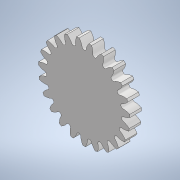
# Autodesk Inventor part: Pinion222
Saved by Autodesk Inventor 2022 (Build 260153000, 153)
## iProperties
Created: 2022-06-04
Part Number: Pinion222
Material: Generic
Document SubType Name: Modeling
Designer: frede
Density: 1 g/cm^3
Appearance: Default
Author: frede
Autodesk Inventor part; units mm, degrees
ref_plane "YZ Plane" through (0, 0, 0) normal (1, 0, 0) x (0, 1, 0)
ref_plane "XZ Plane" through (0, 0, 0) normal (0, 1, 0) x (-1, 0, 0)
ref_plane "XY Plane" through (0, 0, 0) normal (0, 0, 1) x (1, 0, 0)
sketch "Sketch1" plane through (0, 0, 0) normal (0, 0, 1) x (1, 0, 0)
  spline S0 degree 3 poles (-3.3489, 31.0344) (-3.2669, 30.9208) (-3.1027, 30.6937) (-2.8692, 30.344) (-2.6455, 29.988) (-2.4333, 29.625) (-2.2335, 29.255) (-2.0474, 28.8779) (-1.8767, 28.4936) (-1.7233, 28.102) (-1.5918, 27.7027) (-1.4824, 27.296) (-1.4363, 26.9482) (-1.3713, 26.6753) (-1.3031, 26.4761) (-1.2148, 26.2851) (-1.1055, 26.1048) (-0.9893, 25.973) (-0.8874, 25.8765) (-0.8022, 25.8147) (-0.714, 25.7572) (-0.6186, 25.7128) (-0.5212, 25.6728) (-0.4188, 25.6481) (-0.3154, 25.6283) (-0.1751, 25.6229) (0, 25.6264) (0.1751, 25.6229) (0.3154, 25.6283) (0.4188, 25.6481) (0.5212, 25.6728) (0.6186, 25.7128) (0.714, 25.7572) (0.8022, 25.8147) (0.8874, 25.8765) (0.9893, 25.973) (1.1055, 26.1048) (1.2148, 26.2851) (1.3031, 26.4761) (1.3713, 26.6753) (1.4363, 26.9482) (1.4824, 27.296) (1.5918, 27.7027) (1.7233, 28.102) (1.8767, 28.4936) (2.0474, 28.8779) (2.2335, 29.255) (2.4333, 29.625) (2.6455, 29.988) (2.8692, 30.344) (3.1027, 30.6937) (3.2669, 30.9208) (3.3489, 31.0344) knots 0 0 0 0 0.042039 0.084079 0.126119 0.168158 0.210197 0.252236 0.294274 0.336311 0.378346 0.420376 0.46241 0.483428 0.504444 0.525453 0.546459 0.567453 0.577965 0.588475 0.598984 0.609494 0.620001 0.63051 0.641019 0.651526 0.672547 0.693567 0.704074 0.714583 0.725092 0.735599 0.746109 0.756618 0.767128 0.77764 0.798635 0.81964 0.840649 0.861665 0.882683 0.924717 0.966747 1.008782 1.050819 1.092857 1.134896 1.176935 1.218975 1.261014 1.303054 1.345093 1.345093 1.345093 1.345093
  circle A0 centre (0, 0) radius 25.625 construction
  circle A1 centre (0, 0) radius 27.0162 construction
  circle A2 centre (0, 0) radius 28.75 construction
  circle A3 centre (0, 0) radius 31.2146
  point P0 (-3.1048, 30.6922)
  point P1 (-2.8708, 30.3429)
  point P2 (-2.6474, 29.9868)
  point P3 (-2.4354, 29.6238)
  point P4 (-2.2358, 29.2538)
  point P5 (-2.05, 28.8767)
  point P6 (-1.8796, 28.4924)
  point P7 (-1.7269, 28.1007)
  point P8 (-1.5955, 27.7015)
  point P9 (-1.4914, 27.2943)
  point P10 (-1.4177, 26.8804)
  point P11 (-1.368, 26.6762)
  point P12 (-1.2997, 26.4774)
  point P13 (-1.2113, 26.2869)
  point P14 (-1.1005, 26.1085)
  point P15 (-0.9631, 25.9497)
  point P16 (-0.8859, 25.8783)
  point P17 (-0.8017, 25.8154)
  point P18 (-0.7128, 25.7594)
  point P19 (-0.6182, 25.7135)
  point P20 (-0.5203, 25.6754)
  point P21 (-0.4186, 25.6489)
  point P22 (-0.3151, 25.6309)
  point P23 (-0.2102, 25.6249)
  point P24 (0, 25.625)
  point P25 (0.2102, 25.6249)
  point P26 (0.3151, 25.6309)
  point P27 (0.4186, 25.6489)
  point P28 (0.5203, 25.6754)
  point P29 (0.6182, 25.7135)
  point P30 (0.7128, 25.7594)
  point P31 (0.8017, 25.8154)
  point P32 (0.8859, 25.8783)
  point P33 (0.9631, 25.9497)
  point P34 (1.1005, 26.1085)
  point P35 (1.2113, 26.2869)
  point P36 (1.2997, 26.4774)
  point P37 (1.368, 26.6762)
  point P38 (1.4177, 26.8804)
  point P39 (1.4914, 27.2943)
  point P40 (1.5955, 27.7015)
  point P41 (1.7269, 28.1007)
  point P42 (1.8796, 28.4924)
  point P43 (2.05, 28.8767)
  point P44 (2.2358, 29.2538)
  point P45 (2.4354, 29.6238)
  point P46 (2.6474, 29.9868)
  point P47 (2.8708, 30.3429)
  point P48 (3.1048, 30.6922)
  constraints: 4 centre point, 2 point on circle, 107 other
extrude "Extrusion1" add sketch "Sketch1" against normal blind 8
extrude "Extrusion2" cut sketch "Sketch1" against normal through all contours A3 S0 picked at (-0.4102, 29.7407)
pattern_circular "Circular Pattern1" count 23 over 360 about axis through (0, 0, 0) along (0, 0, -1) of "Extrusion2"
sketch "Sketch2" plane through (0, 0, 0) normal (0, 0, 1) x (1, 0, 0)
  arc A0 (-47.6633, 66.2169) -> (-53.0859, 65.6856) centre (-50.338, 65.578) ccw projected
  line L0 (-53.0859, 65.6856) -> (-53.5665, 53.4075) projected
  arc A1 (-53.5665, 53.4075) -> (-52.7565, 45.1423) centre (-48.7825, 49.704) ccw projected
  line L1 (-52.7565, 45.1423) -> (-49.9016, 33.1911) projected
  arc A2 (-49.9016, 33.1911) -> (-44.479, 33.7225) centre (-47.2269, 33.8301) ccw projected
  line L2 (-44.479, 33.7225) -> (-43.9985, 46.0006) projected
  arc A3 (-43.9985, 46.0006) -> (-44.8084, 54.2658) centre (-48.7825, 49.704) ccw projected
  line L3 (-44.8084, 54.2658) -> (-47.6633, 66.2169) projected
  circle A4 centre (-48.7825, 49.704) radius 4.4 projected
  circle A5 centre (-48.0998, 42.7374) radius 0.75 projected
  circle A6 centre (-47.8072, 39.7517) radius 0.75 projected
  circle A7 centre (-47.5146, 36.766) radius 0.75 projected
  circle A8 centre (-50.3429, 65.6278) radius 0.75 projected
  circle A9 centre (-50.0503, 62.6421) radius 0.75 projected
  circle A10 centre (-49.7577, 59.6564) radius 0.75 projected
  circle A11 centre (-47.222, 33.7803) radius 0.75 projected
  circle A12 centre (-49.4651, 56.6707) radius 0.75 projected
  arc A13 (1.1192, 16.5129) -> (-4.3035, 15.9815) centre (-1.5556, 15.874) ccw
  line L4 (-4.3035, 15.9815) -> (-4.784, 3.7035)
  arc A14 (-4.784, 3.7035) -> (-3.974, -4.5617) centre (0, 0) ccw
  line L5 (-3.974, -4.5617) -> (-1.1192, -16.5129)
  arc A15 (4.784, -3.7035) -> (3.974, 4.5617) centre (0, 0) ccw
  line L6 (3.974, 4.5617) -> (1.1192, 16.5129)
  arc A16 (-1.1192, -16.5129) -> (4.3035, -15.9815) centre (1.5556, -15.874) ccw
  line L7 (4.3035, -15.9815) -> (4.784, -3.7035)
  line L8 (-3.974, -4.5617) -> (-1.1192, -16.5129)
  line L9 (-1.6055, -16.6291) -> (-4.424, -4.8302)
  arc A17 (-5.2775, 3.8795) -> (-4.424, -4.8302) centre (0, 0) ccw
  line L10 (-5.2775, 3.8795) -> (-4.8031, 16.0011)
  arc A18 (1.6055, 16.6291) -> (-4.8031, 16.0011) centre (-1.5556, 15.874) ccw
  line L11 (1.6055, 16.6291) -> (4.424, 4.8302)
  arc A19 (5.1794, -4.0096) -> (4.424, 4.8302) centre (0, 0) ccw
  line L12 (5.2836, -3.723) -> (4.8031, -16.0011)
  arc A20 (-1.6055, -16.6291) -> (4.8031, -16.0011) centre (1.5556, -15.874) ccw
  point P0 (-1.1192, -16.5129)
  point P1 (4.784, -3.7035)
  point P2 (1.1192, 16.5129)
  point P3 (5.2775, -3.8795)
  dimension "d9" = 360
  dimension "d13" = 0.5
  dimension "d14" = 0.5
  dimension "d15" = 0.5
  constraints: 18 end point, 16 point on circle, 8 centre point, 2 coincident, 24 other
  measures "d13" distance between parallel lines of L4 L10
  measures "d14" distance between parallel lines of L6 L11
  measures "d15" distance between parallel lines of L7 L12
extrude "Extrusion3" cut sketch "Sketch2" against normal blind 2.5 contours L6 A15 L7 A16 L5 A14 L4 A13 | L9 A17 L10 A18 L11 A19 L12 A20
sketch "Sketch3" plane through (0, 0, 0) normal (0, 0, 1) x (1, 0, 0)
  circle A0 centre (0, 0) radius 2
  dimension "d16" = 4
  constraints: 1 centre point, 1 coincident
  measures "d16" diameter of A0
extrude "Extrusion4" cut sketch "Sketch3" against normal through all
equation "\"d0\" = FaceWidth"
equation "\"Module\" = 2.5"
equation "\"PressureAngle\" = 20deg"
equation "\"UnitProfileClearance\" = 0.25"
equation "\"UnitRoundRadius\" = 0.35"
equation "\"HeadDiameter\" = 62.42917"
equation "\"RootDiameter\" = 51.25"
equation "\"BaseDiameter\" = 54.03233"
equation "\"PitchDiameter\" = 57.5"
equation "\"FaceWidth\" = 8"
equation "\"HelixAngle\" = 0"
equation "\"UnitCorrection\" = 0"
equation "\"UnitAddendumModification\" = 0.014165"
equation "\"CircularPitch\" = 7.853982"
equation "\"UnitBacklashShift\" = 0"
equation "\"TotalToolShift\" = 0"
equation "\"IsInternal\" = 0"
body "Solid1"
